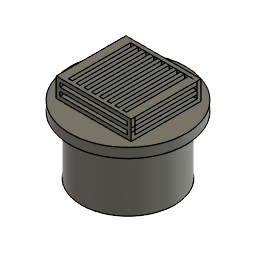
Cold outlet (Autodesk Fusion 360 design; units mm, degrees)
Autodesk Fusion 360 part; units mm, degrees
sketch "Sketch1" plane through (0, 0, 0) normal (0, 0, 1) x (1, 0, 0) in component "sleeve v2 v1"
  circle A0 centre (0, 0) radius 30
  dimension "d1" = 60
  constraint coincident A0.centre origin
  measures "d1" diameter of A0
extrude "Extrude1" add sketch "Sketch1" along normal blind 5 makes body 1 in component "sleeve v2 v1"
sketch "Sketch2" plane through (0, 0, 5) normal (0, 0, 1) x (-1, 0, 0) in component "sleeve v2 v1"
  circle A0 centre (0, 0) radius 30
  circle A1 centre (0, 0) radius 24.1
  dimension "d4" = 48.2
  constraint coincident A0.centre A1.centre
  measures "d4" diameter of A1
extrude "Extrude2" add sketch "Sketch2" along normal blind 25 contours A1 bodies 1 in component "sleeve v2 v1"
sketch "Sketch3" plane through (0, 0, 0) normal (0, 0, -1) x (1, 0, 0) in component "sleeve v2 v1"
  circle A0 centre (0, 0) radius 30
  circle A1 centre (0, 0) radius 24.1
extrude "Extrude3" add sketch "Sketch3" along normal blind 30 contours A1 bodies 1 in component "sleeve v2 v1"
sketch "Sketch4" plane through (0, 0, 30) normal (0, 0, 1) x (-1, 0, 0) in component "sleeve v2 v1"
  circle A0 centre (0, 0) radius 24.1
  circle A1 centre (0, 0) radius 21.1
  dimension "d9" = -3
extrude "Extrude4" cut sketch "Sketch4" against normal blind 60 contours A1 bodies 1 in component "sleeve v2 v1"
extrude "Extrude7" cut 1 faces at (-23.0103, 1.1973, 30) along direction (0, 0, -1) blind 15 on bodies 1 bodies 1 in component "sleeve v2 v1"
extrude "Extrude8" cut 1 faces at (-23.0103, 1.1973, 15) along direction (0, 0, -1) blind 10 on bodies 1 bodies 1 in component "sleeve v2 v1"
sketch "Sketch3 (2)" plane through (0, 4.7273, 0) normal (0, 1, 0) x (-1, 0, 0)
  circle A0 centre (0, 0.2727) radius 21.1
  circle A1 centre (0, 0.2727) radius 30
  circle A2 centre (0, 0) radius 26.5
  line L0 (-19.3899, 18.0632) -> (19.3899, 18.0632)
  line L1 (19.3899, 18.0632) -> (19.3899, -18.0632)
  line L2 (19.3899, -18.0632) -> (-19.3899, -18.0632)
  line L3 (-19.3899, -18.0632) -> (-19.3899, 18.0632)
  line L4 (-19.3899, 18.0632) -> (19.3899, -18.0632) construction
  line L5 (19.3899, 18.0632) -> (-19.3899, -18.0632) construction
  line L6 (-14.3899, 13.0632) -> (14.3899, 13.0632)
  line L7 (14.3899, 13.0632) -> (14.3899, -13.0632)
  line L8 (14.3899, -13.0632) -> (-14.3899, -13.0632)
  line L9 (-14.3899, -13.0632) -> (-14.3899, 13.0632)
  dimension "d67" = 53
  dimension "d68" = 5
  constraint coincident A2.centre origin
  constraint horizontal L0
  constraint perpendicular L0 L1
  constraint parallel L0 L2
  constraint parallel L1 L3
  constraint coincident L4 A2.centre
  constraint coincident L5 A2.centre
  constraint coincident A2 L0.start
  measures "d67" diameter of A2
extrude "Extrude2'" add sketch "Sketch3 (2)" along normal blind 10 separate body contours A0 L0 L1 L2 L3 | A0 L0 L1 | A0 L1 L2 | A0 L0 L3 | A0 L2 L3 makes body 2
sketch "Sketch4 (2)" plane through (0, 4.7273, 0) normal (0, 1, 0) x (-1, 0, 0)
  circle A0 centre (0, 0.2727) radius 21.1
  circle A1 centre (0, 0.2727) radius 30
extrude "Extrude9" add sketch "Sketch4 (2)" against normal blind 5 contours A0 sketch seen with x (1, 0, 0) y (0, 0, 1) z (0, -1, 0) at (0, 0.2727, 0.2727) bodies 1 in component "sleeve v2 v1"
sketch "Sketch5" plane through (0, 14.7273, 0) normal (0, 1, 0) x (-1, 0, 0)
  line L0 (14.3899, -13.0632) -> (-14.3899, -13.0632)
  line L1 (-14.3899, -13.0632) -> (-14.3899, 13.0632)
  line L2 (-14.3899, 13.0632) -> (14.3899, 13.0632)
  line L3 (14.3899, 13.0632) -> (14.3899, -13.0632)
  line L4 (-19.3899, -18.0632) -> (19.3899, -18.0632)
  line L5 (19.3899, -18.0632) -> (19.3899, 18.0632)
  line L6 (19.3899, 18.0632) -> (-19.3899, 18.0632)
  line L7 (-19.3899, 18.0632) -> (-19.3899, -18.0632)
extrude "Extrude10" cut sketch "Sketch5" against normal blind 15 contours L0 L1 L2 L3 sketch seen with x (1, 0, 0) y (0, 0, 1) z (0, -1, 0) at (0, 0.2727, 0.2727) bodies 1 in component "sleeve v2 v1"
sketch "Sketch6" plane through (19.3899, 0, 0) normal (1, 0, 0) x (0, 0, -1)
  line L0 (-18.0632, 4.7273) -> (18.0632, 4.7273)
  line L1 (18.0632, 4.7273) -> (18.0632, 14.7273)
  line L2 (18.0632, 14.7273) -> (-18.0632, 14.7273)
  line L3 (-18.0632, 14.7273) -> (-18.0632, 4.7273)
  line L4 (16.0632, 6.7273) -> (16.0632, 12.7273)
  line L5 (16.0632, 12.7273) -> (-16.0632, 12.7273)
  line L6 (-16.0632, 12.7273) -> (-16.0632, 6.7273)
  line L7 (-16.0632, 6.7273) -> (16.0632, 6.7273)
  dimension "d75" = -2
extrude "Extrude3'" cut sketch "Sketch6" against normal blind 38.78 contours L4 L5 L6 L7 bodies 2
sketch "Sketch7" plane through (0, 0, -18.0632) normal (0, 0, -1) x (-1, 0, 0)
  line L0 (-19.3899, 4.7273) -> (19.3899, 4.7273)
  line L1 (19.3899, 4.7273) -> (19.3899, 14.7273)
  line L2 (19.3899, 14.7273) -> (-19.3899, 14.7273)
  line L3 (-19.3899, 14.7273) -> (-19.3899, 4.7273)
  line L4 (-17.3899, 6.7273) -> (17.3899, 6.7273)
  line L5 (17.3899, 6.7273) -> (17.3899, 12.7273)
  line L6 (17.3899, 12.7273) -> (-17.3899, 12.7273)
  line L7 (-17.3899, 12.7273) -> (-17.3899, 6.7273)
  dimension "d78" = -2
extrude "Extrude4'" cut sketch "Sketch7" against normal blind 36.1265 contours L4 L5 L6 L7 bodies 2
sketch "Sketch8" plane through (0, 14.7273, 0) normal (0, 1, 0) x (-1, 0, 0)
  line L0 (14.3899, -13.0632) -> (-14.3899, -13.0632)
  line L1 (-14.3899, -13.0632) -> (-14.3899, 13.0632)
  line L2 (-14.3899, 13.0632) -> (14.3899, 13.0632)
  line L3 (14.3899, 13.0632) -> (14.3899, -13.0632)
  line L4 (-19.3899, -18.0632) -> (19.3899, -18.0632)
  line L5 (19.3899, -18.0632) -> (19.3899, 18.0632)
  line L6 (19.3899, 18.0632) -> (-19.3899, 18.0632)
  line L7 (-19.3899, 18.0632) -> (-19.3899, -18.0632)
  line L8 (17.3899, 16.0632) -> (-17.3899, 16.0632)
  line L9 (-17.3899, 16.0632) -> (-17.3899, -16.0632)
  line L10 (-17.3899, -16.0632) -> (17.3899, -16.0632)
  line L11 (17.3899, -16.0632) -> (17.3899, 16.0632)
  dimension "d81" = -2
extrude "Extrude5" cut sketch "Sketch8" against normal blind 15 contours L8 L9 L10 L11 bodies 2
sketch "Sketch9" plane through (0, 0, 18.0632) normal (0, 0, 1) x (1, 0, 0)
  line L0 (17.3899, 6.7273) -> (-17.3899, 6.7273)
  line L1 (-17.3899, 6.7273) -> (-17.3899, 12.7273)
  line L2 (-17.3899, 12.7273) -> (17.3899, 12.7273)
  line L3 (17.3899, 12.7273) -> (17.3899, 6.7273)
  line L4 (-19.3899, 4.7273) -> (19.3899, 4.7273)
  line L5 (19.3899, 4.7273) -> (19.3899, 14.7273)
  line L6 (19.3899, 14.7273) -> (-19.3899, 14.7273)
  line L7 (-19.3899, 14.7273) -> (-19.3899, 4.7273)
  line L8 (-1, 14.7273) -> (1, 14.7273)
  line L9 (1, 14.7273) -> (1, 12.7273)
  line L10 (1, 12.7273) -> (-1, 12.7273)
  line L11 (-1, 12.7273) -> (-1, 14.7273)
  line L12 (5, 12.7273) -> (3, 12.7273)
  line L13 (5, 14.7273) -> (5, 12.7273)
  line L14 (3, 14.7273) -> (5, 14.7273)
  line L15 (3, 12.7273) -> (3, 14.7273)
  line L16 (-3, 12.7273) -> (-5, 12.7273)
  line L17 (-3, 14.7273) -> (-3, 12.7273)
  line L18 (-5, 14.7273) -> (-3, 14.7273)
  line L19 (-5, 12.7273) -> (-5, 14.7273)
  line L20 (11, 12.7273) -> (11, 14.7273)
  line L21 (7, 14.7273) -> (9, 14.7273)
  line L22 (15, 12.7273) -> (15, 14.7273)
  line L23 (11, 14.7273) -> (13, 14.7273)
  line L24 (17, 12.7273) -> (15, 12.7273)
  line L25 (13, 12.7273) -> (11, 12.7273)
  line L26 (13, 14.7273) -> (13, 12.7273)
  line L27 (7, 12.7273) -> (7, 14.7273)
  line L28 (9, 12.7273) -> (7, 12.7273)
  line L29 (17, 14.7273) -> (17, 12.7273)
  line L30 (9, 14.7273) -> (9, 12.7273)
  line L31 (15, 14.7273) -> (17, 14.7273)
  line L32 (-17, 14.7273) -> (-15, 14.7273)
  line L33 (-15, 14.7273) -> (-15, 12.7273)
  line L34 (-7, 12.7273) -> (-9, 12.7273)
  line L35 (-11, 14.7273) -> (-11, 12.7273)
  line L36 (-13, 14.7273) -> (-11, 14.7273)
  line L37 (-17, 12.7273) -> (-17, 14.7273)
  line L38 (-15, 12.7273) -> (-17, 12.7273)
  line L39 (-9, 14.7273) -> (-7, 14.7273)
  line L40 (-11, 12.7273) -> (-13, 12.7273)
  line L41 (-7, 14.7273) -> (-7, 12.7273)
  line L42 (-13, 12.7273) -> (-13, 14.7273)
  line L43 (-9, 12.7273) -> (-9, 14.7273)
  dimension "d84" = 2
  dimension "d85" = 2
  dimension "d86" = 2
  dimension "d87" = 2
  dimension "d88" = 2
  dimension "d89" = 2
  dimension "d90" = 2
  dimension "d91" = 2
  dimension "d92" = 2
  constraint horizontal L8
  constraint vertical L9
  constraint horizontal L10
  constraint vertical L11
  constraint coincident L2 L9.end
  constraint coincident L6 L8.start
  constraint midpoint L2 L10
  constraint horizontal L14
  constraint vertical L13
  constraint horizontal L12
  constraint vertical L15
  constraint horizontal L18
  constraint vertical L17
  constraint horizontal L16
  constraint vertical L19
  constraint horizontal L23
  constraint vertical L26
  constraint horizontal L25
  constraint vertical L20
  constraint horizontal L31
  constraint vertical L29
  constraint horizontal L24
  constraint vertical L22
  constraint horizontal L21
  constraint vertical L30
  constraint horizontal L28
  constraint vertical L27
  constraint horizontal L36
  constraint vertical L35
  constraint horizontal L40
  constraint vertical L42
  constraint horizontal L39
  constraint vertical L41
  constraint horizontal L34
  constraint vertical L43
  constraint horizontal L32
  constraint vertical L33
  constraint horizontal L38
  constraint vertical L37
  measures "d84" distance of L9 L11
  measures "d85" distance of L13 L15
  measures "d86" distance of L17 L19
  measures "d87" distance of L20 L26
  measures "d88" distance of L22 L29
  measures "d89" distance of L27 L30
  measures "d90" distance of L35 L42
  measures "d91" distance of L41 L43
  measures "d92" distance of L33 L37
extrude "Extrude6" add sketch "Sketch9" against normal blind 34.126 contours L2 L6 L22 L24 L29 L31 | L2 L6 L32 L33 L37 L38 | L2 L6 L20 L23 L25 L26 | L2 L6 L35 L36 L40 L42 | L2 L6 L21 L27 L28 L30 | L2 L6 L34 L39 L41 L43 | L2 L6 L12 L13 L14 L15 | L2 L6 L16 L17 L18 L19 | L2 L6 L8 L9 L10 L11 bodies 2
extrude "Extrude7'" add 1 faces at (17, 14.0606, 5.3546) along direction (1, 0, 0) blind 2.39 on bodies 2 bodies 2
extrude "Extrude8'" add 1 faces at (-17.3899, 14.0606, 5.3544) along direction (1, 0, 0) blind 2.39 on bodies 2 bodies 2
sketch "Sketch10" plane through (-17.3899, 0, 0) normal (1, 0, 0) x (0, 0, -1)
  line L0 (-16.0632, 6.7273) -> (-16.0632, 12.7273)
  line L1 (-16.0632, 12.7273) -> (-18.0632, 12.7273)
  line L2 (-18.0632, 12.7273) -> (-18.0632, 6.7273)
  line L3 (-18.0632, 6.7273) -> (-16.0632, 6.7273)
  line L4 (-18.0632, 10.7273) -> (-16.0632, 10.7273)
  line L5 (-16.0632, 10.7273) -> (-16.0632, 8.7273)
  line L6 (-16.0632, 8.7273) -> (-18.0632, 8.7273)
  line L7 (-18.0632, 8.7273) -> (-18.0632, 10.7273)
  dimension "d99" = 2
  constraint horizontal L4
  constraint vertical L5
  constraint horizontal L6
  constraint vertical L7
  constraint coincident L2 L4.start
  constraint midpoint L0 L5
  measures "d99" distance of L4.start L6.end
extrude "Extrude9'" add sketch "Sketch10" along normal blind 36.78 contours L0 L2 L4 L5 L6 L7 bodies 2
sketch "Sketch11" plane through (0, 0, 16.0632) normal (0, 0, -1) x (-1, 0, 0)
  line L0 (17.3899, 12.7273) -> (17.3899, 10.7273)
  line L1 (17.3899, 10.7273) -> (-17.3899, 10.7273)
  line L2 (-17.3899, 10.7273) -> (-17.3899, 12.7273)
  line L3 (-17.3899, 12.7273) -> (-19.3899, 12.7273)
  line L4 (-19.3899, 12.7273) -> (-19.3899, 10.7273)
  line L5 (-19.3899, 10.7273) -> (-19.3901, 10.7273)
  line L6 (-19.3901, 10.7273) -> (-19.3901, 8.7273)
  line L7 (-19.3901, 8.7273) -> (-19.3899, 8.7273)
  line L8 (-19.3899, 8.7273) -> (-19.3899, 6.7273)
  line L9 (-19.3899, 6.7273) -> (-17.3899, 6.7273)
  line L10 (-17.3899, 6.7273) -> (-17.3899, 8.7273)
  line L11 (-17.3899, 8.7273) -> (17.3899, 8.7273)
  line L12 (17.3899, 8.7273) -> (17.3899, 6.7273)
  line L13 (17.3899, 6.7273) -> (19.3899, 6.7273)
  line L14 (19.3899, 6.7273) -> (19.3899, 12.7273)
  line L15 (19.3899, 12.7273) -> (17.3899, 12.7273)
  line L16 (-19.3899, 10.7273) -> (-17.3899, 10.7273)
  line L17 (-17.3899, 10.7273) -> (-17.3899, 8.7273)
  line L18 (-17.3899, 8.7273) -> (-19.3899, 8.7273)
  line L19 (-19.3899, 8.7273) -> (-19.3899, 10.7273)
  constraint horizontal L16
  constraint vertical L17
  constraint horizontal L18
  constraint vertical L19
  constraint coincident L10.end L11.start
  constraint coincident L4.end L5.start
extrude "Extrude10'" add sketch "Sketch11" along normal blind 32.126 contours L6 L16 L17 L18 L19 bodies 2
sketch "Sketch12" plane through (17.3899, 0, 0) normal (-1, 0, 0) x (0, 0, 1)
  line L0 (-16.0632, 6.7273) -> (-16.0632, 12.7273)
  line L1 (-16.0632, 12.7273) -> (-18.0632, 12.7273)
  line L2 (-18.0632, 12.7273) -> (-18.0632, 6.7273)
  line L3 (-18.0632, 6.7273) -> (-16.0632, 6.7273)
  line L4 (-18.0632, 10.7273) -> (-16.0632, 10.7273)
  line L5 (-16.0632, 10.7273) -> (-16.0632, 8.7273)
  line L6 (-16.0632, 8.7273) -> (-18.0632, 8.7273)
  line L7 (-18.0632, 8.7273) -> (-18.0632, 10.7273)
  dimension "d104" = 2
  dimension "d105" = 2
  constraint horizontal L4
  constraint vertical L5
  constraint horizontal L6
  constraint vertical L7
  constraint coincident L2 L4.start
  constraint midpoint L0 L5
  measures "d104" distance of L4.start L4.end
  measures "d105" distance of L4.start L6.end
extrude "Extrude11" add sketch "Sketch12" along normal blind 34.78 contours L0 L2 L4 L5 L6 L7 bodies 2
sketch "Sketch13" plane through (0, 0, -16.0632) normal (0, 0, 1) x (1, 0, 0)
  line L0 (17.3899, 12.7273) -> (17.3899, 10.7273)
  line L1 (17.3899, 10.7273) -> (-17.3899, 10.7273)
  line L2 (-17.3899, 10.7273) -> (-17.3899, 12.7273)
  line L3 (-17.3899, 12.7273) -> (-19.3899, 12.7273)
  line L4 (-19.3899, 12.7273) -> (-19.3899, 6.7273)
  line L5 (-19.3899, 6.7273) -> (-17.3899, 6.7273)
  line L6 (-17.3899, 6.7273) -> (-17.3899, 8.7273)
  line L7 (-17.3899, 8.7273) -> (17.3899, 8.7273)
  line L8 (17.3899, 8.7273) -> (17.3899, 6.7273)
  line L9 (17.3899, 6.7273) -> (19.3899, 6.7273)
  line L10 (19.3899, 6.7273) -> (19.3899, 12.7273)
  line L11 (19.3899, 12.7273) -> (17.3899, 12.7273)
  line L12 (-17.3899, 10.7273) -> (-19.3899, 10.7273)
  line L13 (-19.3899, 10.7273) -> (-19.3899, 8.7273)
  line L14 (-19.3899, 8.7273) -> (-17.3899, 8.7273)
  line L15 (-17.3899, 8.7273) -> (-17.3899, 10.7273)
  dimension "d108" = 2
  constraint horizontal L12
  constraint vertical L13
  constraint horizontal L14
  constraint vertical L15
  constraint coincident L1.end L2.start
  measures "d108" distance of L1.end L6.end
extrude "Extrude12" add sketch "Sketch13" along normal blind 34.126 contours L4 L12 L13 L14 L15 bodies 2
extrude "Extrude5'" [suppressed] in component "sleeve v2 v1"
extrude "Extrude6'" [suppressed] in component "sleeve v2 v1"
sketch "Sketch1 (2)" plane through (0, -0.2727, 0) normal (0, 1, 0) x (-1, 0, 0)
  circle A0 centre (0, 0.2727) radius 24.1
  circle A1 centre (0, 0.2727) radius 21.1
  line L0 (-27.5, 27.5) -> (27.5, 27.5)
  line L1 (27.5, 27.5) -> (27.5, -27.5)
  line L2 (27.5, -27.5) -> (-27.5, -27.5)
  line L3 (-27.5, -27.5) -> (-27.5, 27.5)
  line L4 (-27.5, 27.5) -> (27.5, -27.5) construction
  line L5 (27.5, 27.5) -> (-27.5, -27.5) construction
  dimension "d16" = 55
  dimension "d17" = 55
  constraint horizontal L0
  constraint perpendicular L0 L1
  constraint parallel L0 L2
  constraint parallel L1 L3
  constraint coincident L4 origin
  constraint coincident L5 origin
  measures "d16" distance of L1.end L2.end
  measures "d17" distance of L0.end L1.end
extrude "Extrude1'" [suppressed]
sketch "Sketch2 (2)" plane through (0, 9.7273, 0) normal (0, 1, 0) x (-1, 0, 0)
  line L0 (-27.5, -27.5) -> (27.5, -27.5)
  line L1 (27.5, 27.5) -> (-27.5, 27.5)
  line L2 (1, 26.5) -> (-1, 26.5)
  line L3 (-1, 26.5) -> (-1, -26.5)
  line L4 (-1, -26.5) -> (1, -26.5)
  line L5 (1, -26.5) -> (1, 26.5)
  line L6 (1, 26.5) -> (-1, -26.5) construction
  line L7 (-1, 26.5) -> (1, -26.5) construction
  line L8 (5, -26.5) -> (5, 26.5)
  line L9 (3, 26.5) -> (3, -26.5)
  line L10 (5, 26.5) -> (3, 26.5)
  line L11 (3, 26.5) -> (5, -26.5) construction
  line L12 (3, -26.5) -> (5, -26.5)
  line L13 (5, 26.5) -> (3, -26.5) construction
  line L14 (-3, -26.5) -> (-3, 26.5)
  line L15 (-5, 26.5) -> (-5, -26.5)
  line L16 (-3, 26.5) -> (-5, 26.5)
  line L17 (-5, 26.5) -> (-3, -26.5) construction
  line L18 (-5, -26.5) -> (-3, -26.5)
  line L19 (-3, 26.5) -> (-5, -26.5) construction
  line L20 (-3, -26.5) -> (-3, 26.5)
  line L21 (5, 26.5) -> (3, 26.5)
  line L22 (-1, -26.5) -> (1, -26.5)
  line L23 (-3, 26.5) -> (-5, -26.5) construction
  line L24 (1, -26.5) -> (1, 26.5)
  line L25 (-5, 26.5) -> (-5, -26.5)
  line L26 (-5, 26.5) -> (-3, -26.5) construction
  line L27 (-5, -26.5) -> (-3, -26.5)
  line L28 (1, 26.5) -> (-1, -26.5) construction
  line L29 (-3, 26.5) -> (-5, 26.5)
  line L30 (-1, 26.5) -> (1, -26.5) construction
  line L31 (3, 26.5) -> (3, -26.5)
  line L32 (3, 26.5) -> (5, -26.5) construction
  line L33 (1, 26.5) -> (-1, 26.5)
  line L34 (3, -26.5) -> (5, -26.5)
  line L35 (-1, 26.5) -> (-1, -26.5)
  line L36 (5, -26.5) -> (5, 26.5)
  line L37 (5, 26.5) -> (3, -26.5) construction
  line L38 (9, -26.5) -> (9, 26.5)
  line L39 (17, 26.5) -> (15, 26.5)
  line L40 (11, -26.5) -> (13, -26.5)
  line L41 (9, 26.5) -> (7, -26.5) construction
  line L42 (13, -26.5) -> (13, 26.5)
  line L43 (7, 26.5) -> (7, -26.5)
  line L44 (7, 26.5) -> (9, -26.5) construction
  line L45 (7, -26.5) -> (9, -26.5)
  line L46 (13, 26.5) -> (11, -26.5) construction
  line L47 (9, 26.5) -> (7, 26.5)
  line L48 (11, 26.5) -> (13, -26.5) construction
  line L49 (15, 26.5) -> (15, -26.5)
  line L50 (15, 26.5) -> (17, -26.5) construction
  line L51 (13, 26.5) -> (11, 26.5)
  line L52 (15, -26.5) -> (17, -26.5)
  line L53 (11, 26.5) -> (11, -26.5)
  line L54 (17, -26.5) -> (17, 26.5)
  line L55 (17, 26.5) -> (15, -26.5) construction
  line L56 (-19, 26.5) -> (-21, -26.5) construction
  line L57 (-9, 26.5) -> (-7, -26.5) construction
  line L58 (-9, -26.5) -> (-7, -26.5)
  line L59 (-25, 26.5) -> (-23, -26.5) construction
  line L60 (-21, 26.5) -> (-19, -26.5) construction
  line L61 (-7, -26.5) -> (-7, 26.5)
  line L62 (-11, 26.5) -> (-13, -26.5) construction
  line L63 (-9, 26.5) -> (-9, -26.5)
  line L64 (-17, 26.5) -> (-17, -26.5)
  line L65 (-19, 26.5) -> (-21, -26.5) construction
  line L66 (-19, -26.5) -> (-19, 26.5)
  line L67 (-25, 26.5) -> (-23, -26.5) construction
  line L68 (-15, -26.5) -> (-15, 26.5)
  line L69 (-7, 26.5) -> (-9, -26.5) construction
  line L70 (-7, 26.5) -> (-9, 26.5)
  line L71 (-21, -26.5) -> (-19, -26.5)
  line L72 (-17, -26.5) -> (-15, -26.5)
  line L73 (-19, 26.5) -> (-21, 26.5)
  line L74 (-25, -26.5) -> (-23, -26.5)
  line L75 (-11, -26.5) -> (-11, 26.5)
  line L76 (-25, -26.5) -> (-23, -26.5)
  line L77 (-13, -26.5) -> (-11, -26.5)
  line L78 (-11, 26.5) -> (-13, 26.5)
  line L79 (-13, 26.5) -> (-13, -26.5)
  line L80 (-21, -26.5) -> (-19, -26.5)
  line L81 (-13, 26.5) -> (-11, -26.5) construction
  line L82 (-23, -26.5) -> (-23, 26.5)
  line L83 (-21, 26.5) -> (-21, -26.5)
  line L84 (-23, 26.5) -> (-25, 26.5)
  line L85 (-23, 26.5) -> (-25, 26.5)
  line L86 (-25, 26.5) -> (-25, -26.5)
  line L87 (-25, 26.5) -> (-25, -26.5)
  line L88 (-19, -26.5) -> (-19, 26.5)
  line L89 (-23, 26.5) -> (-25, -26.5) construction
  line L90 (-23, 26.5) -> (-25, -26.5) construction
  line L91 (-21, 26.5) -> (-19, -26.5) construction
  line L92 (-21, 26.5) -> (-21, -26.5)
  line L93 (-23, -26.5) -> (-23, 26.5)
  line L94 (-15, 26.5) -> (-17, 26.5)
  line L95 (-15, 26.5) -> (-17, -26.5) construction
  line L96 (-17, 26.5) -> (-15, -26.5) construction
  line L97 (-19, 26.5) -> (-21, 26.5)
  line L98 (23, -26.5) -> (25, -26.5)
  line L99 (21, -26.5) -> (21, 26.5)
  line L100 (25, 26.5) -> (23, -26.5) construction
  line L101 (19, -26.5) -> (21, -26.5)
  line L102 (25, 26.5) -> (23, 26.5)
  line L103 (21, 26.5) -> (19, 26.5)
  line L104 (21, 26.5) -> (19, -26.5) construction
  line L105 (23, 26.5) -> (23, -26.5)
  line L106 (25, -26.5) -> (25, 26.5)
  line L107 (19, 26.5) -> (19, -26.5)
  line L108 (23, 26.5) -> (25, -26.5) construction
  line L109 (19, 26.5) -> (21, -26.5) construction
  point P0 (4, 0)
  point P1 (4, 0)
  point P2 (-4, 0)
  point P3 (-4, 0)
  point P4 (-4, 0)
  point P5 (-4, 0)
  point P6 (4, 0)
  point P7 (4, 0)
  point P8 (8, 0)
  point P9 (8, 0)
  point P10 (12, 0)
  point P11 (16, 0)
  point P12 (16, 0)
  point P13 (12, 0)
  point P14 (-20, 0)
  point P15 (-20, 0)
  point P16 (-24, 0)
  point P17 (-24, 0)
  point P18 (-24, 0)
  point P19 (-20, 0)
  point P20 (-20, 0)
  point P21 (-24, 0)
  point P22 (-16, 0)
  point P23 (-16, 0)
  point P24 (-12, 0)
  point P25 (-12, 0)
  point P26 (-8, 0)
  point P27 (-8, 0)
  point P28 (20, 0)
  point P29 (20, 0)
  point P30 (24, 0)
  point P31 (24, 0)
  dimension "d21" = 2
  dimension "d22" = 53
  dimension "d23" = 2
  dimension "d24" = 53
  dimension "d25" = 2
  dimension "d26" = 53
  dimension "d27" = 2
  dimension "d28" = 53
  dimension "d29" = 2
  dimension "d30" = 53
  dimension "d31" = 2
  dimension "d32" = 53
  dimension "d33" = 2
  dimension "d34" = 53
  dimension "d35" = 2
  dimension "d36" = 53
  dimension "d37" = 2
  dimension "d38" = 53
  dimension "d39" = 2
  dimension "d40" = 53
  dimension "d41" = 2
  dimension "d42" = 53
  dimension "d45" = 2
  dimension "d46" = 53
  dimension "d47" = 2
  dimension "d48" = 53
  dimension "d51" = 2
  dimension "d52" = 53
  dimension "d53" = 2
  dimension "d54" = 53
  dimension "d55" = 2
  dimension "d56" = 53
  dimension "d57" = 2
  dimension "d58" = 53
  dimension "d61" = 2
  dimension "d62" = 53
  constraint horizontal L2
  constraint perpendicular L2 L3
  constraint parallel L2 L4
  constraint parallel L3 L5
  constraint coincident L6 origin
  constraint coincident L7 origin
  constraint horizontal L10
  constraint perpendicular L9 L10
  constraint parallel L10 L12
  constraint parallel L8 L9
  constraint coincident P7 L13
  constraint coincident P7 L11
  constraint coincident P7 P6
  constraint horizontal L16
  constraint perpendicular L15 L16
  constraint parallel L16 L18
  constraint parallel L14 L15
  constraint coincident P5 L19
  constraint coincident P5 L17
  constraint coincident P5 P4
  constraint horizontal L33
  constraint perpendicular L33 L35
  constraint parallel L22 L33
  constraint parallel L24 L35
  constraint coincident origin L28
  constraint coincident origin L30
  constraint horizontal L21
  constraint perpendicular L21 L31
  constraint parallel L21 L34
  constraint parallel L31 L36
  constraint coincident P7 L37
  constraint coincident P7 L32
  constraint horizontal L29
  constraint perpendicular L25 L29
  constraint parallel L27 L29
  constraint parallel L20 L25
  constraint coincident P5 L23
  constraint coincident P5 L26
  constraint horizontal L51
  constraint perpendicular L51 L53
  constraint parallel L40 L51
  constraint parallel L42 L53
  constraint coincident P13 L46
  constraint coincident P13 L48
  constraint coincident P13 P10
  constraint horizontal L39
  constraint perpendicular L39 L49
  constraint parallel L39 L52
  constraint parallel L49 L54
  constraint coincident P12 L55
  constraint coincident P12 L50
  constraint coincident P12 P11
  constraint horizontal L47
  constraint perpendicular L43 L47
  constraint parallel L45 L47
  constraint parallel L38 L43
  constraint coincident P9 L41
  constraint coincident P9 L44
  constraint coincident P9 P8
  constraint horizontal L84
  constraint perpendicular L84 L87
  constraint parallel L76 L84
  constraint parallel L87 L93
  constraint coincident P21 L89
  constraint coincident P21 L59
  constraint coincident P21 P18
  constraint horizontal L97
  constraint perpendicular L83 L97
  constraint parallel L80 L97
  constraint parallel L66 L83
  constraint coincident P20 L56
  constraint coincident P20 L60
  constraint coincident P20 P19
  constraint horizontal L85
  constraint perpendicular L85 L86
  constraint parallel L74 L85
  constraint parallel L82 L86
  constraint coincident P21 L90
  constraint coincident P21 L67
  constraint horizontal L73
  constraint perpendicular L73 L92
  constraint parallel L71 L73
  constraint parallel L88 L92
  constraint coincident P20 L65
  constraint coincident P20 L91
  constraint horizontal L78
  constraint perpendicular L78 L79
  constraint parallel L77 L78
  constraint parallel L75 L79
  constraint coincident P25 L62
  constraint coincident P25 L81
  constraint coincident P25 P24
  constraint horizontal L70
  constraint perpendicular L63 L70
  constraint parallel L58 L70
  constraint parallel L61 L63
  constraint coincident P27 L69
  constraint coincident P27 L57
  constraint coincident P27 P26
  constraint horizontal L94
  constraint perpendicular L64 L94
  constraint parallel L72 L94
  constraint parallel L64 L68
  constraint coincident P23 L95
  constraint coincident P23 L96
  constraint coincident P23 P22
  constraint horizontal L102
  constraint perpendicular L102 L105
  constraint parallel L98 L102
  constraint parallel L105 L106
  constraint coincident P31 L100
  constraint coincident P31 L108
  constraint coincident P31 P30
  constraint horizontal L103
  constraint perpendicular L103 L107
  constraint parallel L101 L103
  constraint parallel L99 L107
  constraint coincident P29 L104
  constraint coincident P29 L109
  constraint coincident P29 P28
  measures "d21" distance of L3.end L4.end
  measures "d22" distance of L2.end L3.end
  measures "d23" distance of L9.end L8.start
  measures "d24" distance of L9.end L9.start
  measures "d25" distance of L15.end L14.start
  measures "d26" distance of L15.end L15.start
  measures "d27" distance of L3.end L4.end
  measures "d28" distance of L3.end L2.end
  measures "d29" distance of L9.end L8.start
  measures "d30" distance of L9.end L9.start
  measures "d31" distance of L15.end L14.start
  measures "d32" distance of L15.start L15.end
  measures "d33" distance of L40.start L40.end
  measures "d34" distance of L40.start L48.start
  measures "d35" distance of L49.end L50.end
  measures "d36" distance of L49.end L39.end
  measures "d37" distance of L41.end L38.start
  measures "d38" distance of L43.start L41.end
  measures "d39" distance of L74.start L59.end
  measures "d40" distance of L74.start L59.start
  measures "d41" distance of L56.end L60.end
  measures "d42" distance of L56.end L60.start
  measures "d45" distance of L59.end L74.start
  measures "d46" distance of L59.start L74.start
  measures "d47" distance of L60.end L56.end
  measures "d48" distance of L60.start L56.end
  measures "d51" distance of L62.end L75.start
  measures "d52" distance of L78.end L62.end
  measures "d53" distance of L58.start L57.end
  measures "d54" distance of L58.start L57.start
  measures "d55" distance of L68.start L64.end
  measures "d56" distance of L64.start L64.end
  measures "d57" distance of L98.start L98.end
  measures "d58" distance of L102.end L98.start
  measures "d61" distance of L99.start L101.start
  measures "d62" distance of L103.end L101.start
component "sleeve v2 v1" placed x (1, 0, 0) y (0, 0, -1) z (0, 1, 0) at (0, -0.2727, 0.2727)
